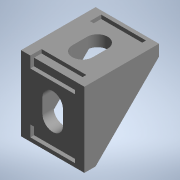
# Autodesk Inventor part: 14056_m
Saved by Autodesk Inventor 2021 (Build 250183000, 183)
## iProperties
Category: PARTsolutions
Company: 8020
Part Number: 14056_m
Material: Generic
Catalog Web Link: www.cadenas.de
Description: 14056, 14051, 14053, 14052, 14054_m-2 Hole Inside Corner Brackets
Vendor: 8020
Document SubType Name: Modeling
Designer: partserver
Manufacturer: 8020
Mass: 2.09215 g
Surface Area: 21.6591 cm^2
Volume: 2.09215 cm^3
Density: 1 g/cm^3
Appearance: PSOLRGB-175-175-175
PSOL_IDENT_0: {$CADENAS_DATA\23d-libs\8020\metric\joining_plates\14056_m.prj},186 {VTYP=3D},{NB=14056_m},{LINA=140
PSOL_IDENT_1: 56},{NN=14056, 14051, 14053, 14052, 14054_m},{DATE=31.07.2020 09:21:28},{GEOMDATE=09.09.2015 07:48:2
PSOL_IDENT_2: 3},{VERSION=},{LINEID=10},{WBVAR=FIN,D},{WBNUMERIC=}  {NB=14056_m},{LINA=14056},{KT=DUMMY},{PN=14056
PSOL_IDENT_3: },{MAT=Die Cast Zinc},{FIN=1},{A=20.00},{B=17.00},{C=5.50},{D=},{D1= '','None','5','5.00' },{D2=0.00
PSOL_IDENT_4: },{T=2.00},{W=.013},{CC=5-20, 6-10, 6-25}
NB: 14056_m
NN: 14056, 14051, 14053, 14052, 14054_m
NT: 2 Hole Inside Corner Brackets
NBSYN: $PN._m
LINA: 14056
CATALOG: 80/20
PN: 14056
MAT: Die Cast Zinc
FIN: Natural
A: 20
B: 17
C: 5.5
T: 2
W: .013
CC: 5-20, 6-10, 6-25
SUPPLIER: 8020
ARTICLENO: 14056_m
BOMINFO: 14056
CREATOR: CADENAS GmbH
Title: 14056
Author: Cadenas PARTsolutions
Comments: 2 Hole Inside Corner Brackets
Autodesk Inventor part; units mm, degrees
ref_plane "YZ Plane" through (0, 0, 0) normal (1, 0, 0) x (0, 1, 0)
ref_plane "XZ Plane" through (0, 0, 0) normal (0, 1, 0) x (-1, 0, 0)
ref_plane "XY Plane" through (0, 0, 0) normal (0, 0, 1) x (1, 0, 0)
sketch "Sketch_1" plane through (0, 0, 0) normal (1, 0, 0) x (0, 1, 0)
  line L0 (0, 20) -> (0, 0)
  line L1 (0, 0) -> (20, 0)
  line L2 (20, 0) -> (20, 3)
  line L3 (20, 3) -> (3, 20)
  line L4 (3, 20) -> (0, 20)
  dimension "d35" = 20
  dimension "d36" = 20
  dimension "d37" = 17
  dimension "d38" = 3
  constraints: 10 end point
  measures "d35" distance of L0.start L0.end
  measures "d36" distance of L0.end L1.end
  measures "d37" horizontal distance of L2.end L3.end
  measures "d38" distance of L1.end L2.end
extrude "Extrusion1" add sketch "Sketch_1" along normal mid plane 17
sketch "Sketch_2" plane through (0, 0, 0) normal (1, 0, 0) x (0, 1, 0)
  line L0 (3, 20) -> (3, 3.5)
  arc A0 (3, 3.5) -> (3.5, 3) centre (3.5, 3.5) ccw
  line L1 (3.5, 3) -> (20, 3)
  line L2 (20, 3) -> (3, 20)
  constraints: 6 end point, 2 point on circle, 1 centre point
extrude "Extrusion2" cut sketch "Sketch_2" along normal mid plane 13
sketch "Sketch_3" plane through (0, 0, 0) normal (1, 0, 0) x (0, 1, 0)
  line L0 (0, 3) -> (0, 0)
  line L1 (0, 0) -> (3, 0)
  line L2 (3, 0) -> (3, 1)
  line L3 (3, 1) -> (1, 1)
  line L4 (1, 1) -> (1, 3)
  line L5 (1, 3) -> (0, 3)
  constraints: 12 end point
extrude "Extrusion3" cut sketch "Sketch_3" along normal mid plane 12
sketch "Sketch_4" plane through (0, 0, 0) normal (1, 0, 0) x (0, 1, 0)
  line L0 (0, 19) -> (0, 16)
  line L1 (0, 16) -> (1, 16)
  line L2 (1, 16) -> (1, 19)
  line L3 (1, 19) -> (0, 19)
  constraints: 8 end point
extrude "Extrusion4" cut sketch "Sketch_4" along normal mid plane 12
sketch "Sketch_5" plane through (0, 0, 0) normal (1, 0, 0) x (0, 1, 0)
  line L0 (16, 1) -> (16, 0)
  line L1 (16, 0) -> (19, 0)
  line L2 (19, 0) -> (19, 1)
  line L3 (19, 1) -> (16, 1)
  constraints: 8 end point
extrude "Extrusion5" cut sketch "Sketch_5" along normal mid plane 12
sketch "Sketch8" plane through (-8.5, 0, 20) normal (0, -1, 0) x (1, 0, 0)
  line L0 (8.5, -8) -> (8.5, -12) construction
  line L1 (5.75, -8) -> (5.75, -12)
  line L2 (11.25, -12) -> (11.25, -8)
  arc A0 (11.25, -8) -> (5.75, -8) centre (8.5, -8) ccw
  arc A1 (5.75, -12) -> (11.25, -12) centre (8.5, -12) ccw
  line L3 (14.5, -20) -> (2.5, -20) projected
  line L4 (17, 0) -> (17, -20) projected
  point P0 (8.5, -20)
  point P1 (8.5, -10)
  dimension "d23" = 2
  dimension "d24" = 5.5
  dimension "d25" = 10
  dimension "d32" = 8.5
  constraints: 8 end point, 4 point on circle, 4 tangent, 2 centre point, 1 midpoint, 1 parallel, 1 vertical
  measures "d23" distance of point (8.5, -10) L0.end
  measures "d24" diameter of A1
  measures "d25" distance from line of L3 point (8.5, -10)
  measures "d32" distance from line of L4 point (8.5, -10)
extrude "Extrusion8" cut sketch "Sketch8" against normal through all
sketch "Sketch9" plane through (8.5, 20, 0) normal (0, 0, -1) x (-1, 0, 0)
  line L0 (8.5, -8) -> (8.5, -12) construction
  line L1 (5.75, -8) -> (5.75, -12)
  line L2 (11.25, -12) -> (11.25, -8)
  arc A0 (11.25, -8) -> (5.75, -8) centre (8.5, -8) ccw
  arc A1 (5.75, -12) -> (11.25, -12) centre (8.5, -12) ccw
  line L3 (17, -20) -> (14.5, -20) projected
  line L4 (0, -20) -> (0, 0) projected
  point P0 (8.5, -20)
  point P1 (8.5, -10)
  dimension "d28" = 2
  dimension "d29" = 5.5
  dimension "d30" = 10
  dimension "d31" = 8.5
  constraints: 8 end point, 4 point on circle, 4 tangent, 2 centre point, 1 midpoint, 1 parallel, 1 vertical
  measures "d28" distance of point (8.5, -10) L0.end
  measures "d29" diameter of A1
  measures "d30" distance from line of L3 point (8.5, -10)
  measures "d31" distance from line of L4 point (8.5, -10)
extrude "Extrusion9" cut sketch "Sketch9" against normal through all
body "Solid1"
